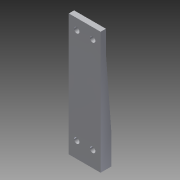
# Autodesk Inventor part: Y_shaft_support_brace_A
Saved by Autodesk Inventor 2013 (Build 170138000, 138)
## iProperties
Created: 2013-09-23
Part Number: Y_shaft_support_brace_A
Material: Aluminum 6061
Document SubType Name: Modeling
Designer: Ian
Density: 2.71 g/cm^3
Mass: 144.593 g
Surface Area: 152.648 cm^2
Volume: 53.3553 cm^3
d0: 4.510 in
d1: 0.750 in
d2: 0.500 in
d3: 1.500 in
d4: 0.500 in
d5: 1.000 in
d6: 0.250 in
d7: 1.500 in
d8: 0.00 deg
d9: 0.375 in
d10: 0.375 in
d11: 0.375 in
d12: 0.375 in
d13: 0.257 in
d20: 0.257 in
d27: 0.250 in
Author: Ian
Autodesk Inventor part; units mm, degrees
ref_plane "YZ Plane" through (0, 0, 0) normal (1, 0, 0) x (0, 1, 0)
ref_plane "XZ Plane" through (0, 0, 0) normal (0, 1, 0) x (-1, 0, 0)
ref_plane "XY Plane" through (0, 0, 0) normal (0, 0, 1) x (1, 0, 0)
sketch "Sketch1" plane through (0, 0, 0) normal (1, 0, 0) x (0, 1, 0)
  line L0 (0, 0) -> (114.554, 0)
  line L1 (0, 0) -> (-19.05, 0)
  line L2 (-19.05, 0) -> (-19.05, -12.7)
  line L3 (-19.05, -12.7) -> (19.05, -12.7)
  line L4 (101.854, -6.35) -> (114.554, -6.35)
  line L5 (114.554, -6.35) -> (127.254, -6.35)
  line L6 (127.254, -6.35) -> (127.254, 0)
  line L7 (127.254, 0) -> (114.554, 0)
  line L8 (114.554, 0) -> (114.554, -6.35) construction
  line L9 (101.854, 0) -> (101.854, -6.35) construction
  line L10 (19.05, -12.7) -> (101.854, -6.35)
  dimension "d0" = 114.554
  dimension "d1" = 19.05
  dimension "d2" = 12.7
  dimension "d3" = 38.1
  dimension "d4" = 12.7
  dimension "d5" = 25.4
  dimension "d6" = 6.35
  constraints: 22 end point, 4 parallel, 3 perpendicular, 2 collinear, 1 horizontal, 1 point on line
  measures "d0" distance of L0.start L0.end
  measures "d1" distance of L0.start L1.end
  measures "d2" distance of L1.end L2.end
  measures "d3" distance of L2.end L3.end
  measures "d4" distance of L4.end L5.end
  measures "d5" distance between parallel lines of L6 L9
  measures "d6" distance of L6.end L5.end
extrude "Extrusion1" add sketch "Sketch1" along normal blind 38.1
sketch "Sketch2" plane through (0, -19.05, -12.7) normal (0, 0, -1) x (-1, 0, 0)
  line L0 (0, 38.1) -> (0, 0) projected
  line L1 (0, 38.1) -> (-38.1, 38.1) projected
  line L2 (-38.1, 0) -> (-38.1, 38.1) projected
  line L3 (0, 0) -> (-38.1, 0) projected
  line L4 (0, 19.05) -> (-38.1, 19.05) construction
  line L5 (-28.575, 38.1) -> (-28.575, 0) construction
  line L6 (-9.525, 38.1) -> (-9.525, 32.2712) construction
  line L7 (-9.525, 32.2712) -> (-9.525, 0) construction
  point P0 (-28.575, 19.05)
  point P1 (-9.525, 19.05)
  dimension "d9" = 9.525
  dimension "d10" = 9.525
  constraints: 8 end point, 6 point on line, 3 perpendicular, 2 midpoint
  measures "d9" distance between parallel lines of L5 L2
  measures "d10" distance between parallel lines of L0 L7
sketch "Sketch3" plane through (0, 101.854, -6.35) normal (0, 0, -1) x (-1, 0, 0)
  line L0 (0, 25.4) -> (0, 0) projected
  line L1 (0, 25.4) -> (-38.1, 25.4) projected
  line L2 (-38.1, 0) -> (-38.1, 25.4) projected
  line L3 (0, 0) -> (-38.1, 0) projected
  line L4 (-38.1, 12.7) -> (0, 12.7) construction
  line L5 (-28.575, 25.4) -> (-28.575, 0) construction
  line L6 (-9.525, 25.4) -> (-9.525, 0) construction
  point P0 (0, -101.854)
  point P1 (-28.575, 12.7)
  point P2 (-9.525, 12.7)
  dimension "d11" = 9.525
  dimension "d12" = 9.525
  constraints: 6 end point, 4 midpoint, 4 point on line, 2 perpendicular
  measures "d11" distance between parallel lines of L2 L5
  measures "d12" distance between parallel lines of L0 L6
hole "Hole1" at (9.525, 0, -12.7) at (28.575, 0, -12.7) direction (0, 0, 1) diameter 6.5278 end through all clearance for "Flat Head Machine Screw (82)" size "1/4" standard "Ansi Unified Screw Threads"
hole "Hole2" at (28.575, 114.554, -6.35) at (9.525, 114.554, -6.35) direction (0, 0, 1) diameter 6.5278 end through all clearance for "Flat Head Machine Screw (82)" size "1/4" standard "Ansi Unified Screw Threads"
fillet_without_effect "Fillet1"
equation "\"d9\" = d10"
equation "\"d12\" = d11"
body "Solid1"
